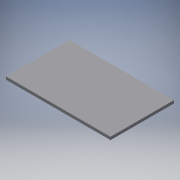
# Autodesk Inventor part: board2
Saved by Autodesk Inventor 2017 (Build 210142000, 142)
## iProperties
Created: 2019-02-06
Part Number: board2
Material: Generic
Document SubType Name: Modeling
Designer: S346559073
Density: 1 g/cm^3
Appearance: Default
Author: S346559073
Autodesk Inventor part; units mm, degrees
ref_plane "YZ Plane" through (0, 0, 0) normal (1, 0, 0) x (0, 1, 0)
ref_plane "XZ Plane" through (0, 0, 0) normal (0, 1, 0) x (-1, 0, 0)
ref_plane "XY Plane" through (0, 0, 0) normal (0, 0, 1) x (1, 0, 0)
sketch "Sketch1" plane through (0, 0, 0) normal (0, 1, 0) x (-1, 0, 0)
  line L0 (0, 0) -> (460.502, 0)
  line L1 (460.502, 0) -> (460.502, 279.4)
  line L2 (460.502, 279.4) -> (0, 279.4)
  line L3 (0, 279.4) -> (0, 0)
  dimension "d0" = 460.502
  dimension "d1" = 279.4
  constraints: 8 end point, 2 parallel, 1 horizontal, 1 perpendicular
  measures "d0" distance of L2.end L1.end
  measures "d1" distance of L1.end L0.end
extrude "Extrusion1" add sketch "Sketch1" along normal blind 12.7
body "Solid1"
